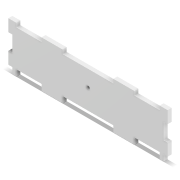
# Autodesk Inventor part: case bottom sides
Saved by Autodesk Inventor 2022.3 (Build 263350030, 350C)
## iProperties
Created: 2021-05-28
Part Number: case bottom sides
Material: ABS Plastic
Document SubType Name: Modeling
Designer: benka
Density: 1.06 g/cm^3
Appearance: Smooth - White
Author: benka
Autodesk Inventor part; units mm, degrees
ref_plane "YZ Plane" through (0, 0, 0) normal (1, 0, 0) x (0, 1, 0)
ref_plane "XZ Plane" through (0, 0, 0) normal (0, 1, 0) x (-1, 0, 0)
ref_plane "XY Plane" through (0, 0, 0) normal (0, 0, 1) x (1, 0, 0)
sketch "Sketch1" plane through (0, 0, 0) normal (0, 0, 1) x (1, 0, 0)
  line L0 (-89.2581, -25.0004) -> (-89.2581, -33.0004)
  line L1 (-89.2581, -25.0004) -> (-58.0081, -25.0004)
  line L2 (-58.0081, -25.0004) -> (-58.0081, -33.0004)
  line L3 (-31.7581, -25.0004) -> (-31.7581, -33.0004)
  line L4 (-31.7581, -25.0004) -> (31.2419, -25.0004)
  line L5 (31.2419, -25.0004) -> (31.2419, -33.0004)
  line L6 (93.7419, -25.0004) -> (98.7419, -25.0004)
  line L7 (98.7419, -25.0004) -> (98.7419, -10.0012)
  line L8 (93.7419, -10.0012) -> (98.7419, -10.0012)
  line L9 (93.7419, -10.0012) -> (93.7419, 9.9988)
  line L10 (93.7419, 9.9988) -> (98.7419, 9.9988)
  line L11 (98.7419, 9.9988) -> (98.7419, 25.0003)
  line L12 (-99.2581, 9.9988) -> (-99.2581, 25.0003)
  line L13 (-99.2581, 9.9988) -> (-94.2581, 9.9988)
  line L14 (-99.2581, -10.0012) -> (-99.2581, -25.0004)
  line L15 (-99.2581, -10.0012) -> (-94.2581, -10.0012)
  line L16 (-99.2581, -25.0004) -> (-94.2581, -25.0004)
  line L17 (-94.2581, 9.9988) -> (-94.2581, -10.0012)
  line L18 (-94.2581, -25.0004) -> (-94.2581, -33.0004)
  line L19 (93.7419, -33.0004) -> (93.7419, -25.0004)
  line L20 (-89.2581, 25.0003) -> (-89.2581, 20.0003)
  line L21 (-89.2581, 20.0003) -> (-58.0081, 20.0003)
  line L22 (-58.0081, 25.0003) -> (-58.0081, 20.0003)
  line L23 (-58.0081, 25.0003) -> (-31.7581, 25.0003)
  line L24 (-31.7581, 25.0003) -> (-31.7581, 20.0003)
  line L25 (-31.7581, 20.0003) -> (31.2419, 20.0003)
  line L26 (31.2419, 25.0003) -> (31.2419, 20.0003)
  line L27 (31.2419, 25.0003) -> (57.4919, 25.0003)
  line L28 (57.4919, 25.0003) -> (57.4919, 20.0003)
  line L29 (57.4919, 20.0003) -> (88.7419, 20.0003)
  line L30 (88.7419, 25.0003) -> (88.7419, 20.0003)
  line L31 (-89.2581, 25.0003) -> (-99.2581, 25.0003)
  line L32 (88.7419, 25.0003) -> (98.7419, 25.0003)
  circle A0 centre (0, 0) radius 2
  line L33 (57.4919, -33.0004) -> (57.4919, -25.0004)
  line L34 (57.4919, -25.0004) -> (88.7419, -25.0004)
  line L35 (88.7419, -25.0004) -> (88.7419, -33.0004)
  line L36 (88.7419, -33.0004) -> (93.7419, -33.0004)
  line L37 (31.2419, -33.0004) -> (57.4919, -33.0004)
  line L38 (-94.2581, -33.0004) -> (-89.2581, -33.0004)
  line L39 (-58.0081, -33.0004) -> (-31.7581, -33.0004)
  point P0 (-93.0453, -16.9364)
  dimension "d46" = 198
  dimension "d47" = 4
  dimension "d48" = 26.25
  dimension "d50" = 63
  dimension "d51" = 31.25
  dimension "d56" = 45.0007
  dimension "d57" = 50.0007
  dimension "d59" = 5
  constraints: 80 end point, 14 vertical, 11 horizontal, 6 perpendicular, 2 collinear, 1 centre point, 1 coincident, 1 point on line, 28 other
  measures "d46" distance between parallel lines of L12 L11
  measures "d47" diameter of A0
  measures "d48" distance between parallel lines of L3 L2
  measures "d50" distance between parallel lines of L3 L5
  measures "d51" distance between parallel lines of L2 L0
  measures "d56" distance between parallel lines of L25 L4
  measures "d57" distance between parallel lines of L4 L27
  measures "d59" distance between parallel lines of L19 L35
extrude "Extrusion3" add sketch "Sketch1" along normal blind 5
body "Solid3"
